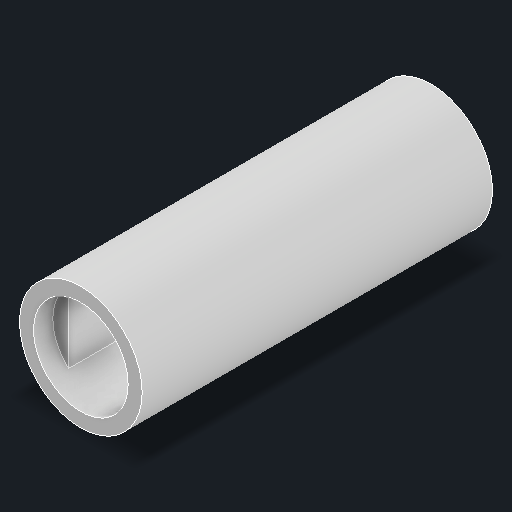
# Autodesk Inventor part: Motor_Lego_Axle_Connector
Saved by Autodesk Inventor 2025 (Build 290162000, 162)
## iProperties
Created: 2024-06-03
Part Number: Motor_Lego_Axle_Connector
Material: Generic
Document SubType Name: Modeling
Designer: Garfieldcmix
Density: 1 g/cm^3
Appearance: Default
Author: Garfieldcmix
Autodesk Inventor part; units mm, degrees
ref_plane "YZ Plane" through (0, 0, 0) normal (1, 0, 0) x (0, 1, 0)
ref_plane "XZ Plane" through (0, 0, 0) normal (0, 1, 0) x (-1, 0, 0)
ref_plane "XY Plane" through (0, 0, 0) normal (0, 0, 1) x (1, 0, 0)
sketch "Motor_Lego_Axle_Connector" plane through (0, 0, 0) normal (0, 0, 1) x (1, 0, 0)
  circle A0 centre (0, 0) radius 3.5
  circle A1 centre (0, 0) radius 2.7
  line L0 (-1.8, 2.0125) -> (-1.8, -2.0125)
  line L1 (0, 3.5) -> (0, -3.5) construction
  line L2 (1.8, 2.0125) -> (1.8, -2.0125)
  line L3 (0.9, 2.4) -> (-0.9, 2.4)
  line L4 (0.9, 2.4) -> (0.9, 1.4)
  line L5 (1.4, 1.4) -> (0.9, 1.4) construction
  line L6 (1.4, 1.4) -> (1.4, 0.9) construction
  arc A2 (0.9, 1.4) -> (1.4, 0.9) centre (1.4, 1.4) ccw
  line L7 (1.4, 0.9) -> (2.4, 0.9)
  line L8 (-0.9, 1.4) -> (-0.9, 2.4)
  arc A3 (-1.4, 0.9) -> (-0.9, 1.4) centre (-1.4, 1.4) ccw
  line L9 (-2.4, 0.9) -> (-1.4, 0.9)
  line L10 (-2.4, 0.9) -> (-2.4, -0.9)
  line L11 (-1.4, -0.9) -> (-2.4, -0.9)
  arc A4 (-0.9, -1.4) -> (-1.4, -0.9) centre (-1.4, -1.4) ccw
  line L12 (-0.9, -2.4) -> (-0.9, -1.4)
  line L13 (-0.9, -2.4) -> (0.9, -2.4)
  line L14 (0.9, -1.4) -> (0.9, -2.4)
  arc A5 (1.4, -0.9) -> (0.9, -1.4) centre (1.4, -1.4) ccw
  line L15 (2.4, -0.9) -> (1.4, -0.9)
  line L16 (2.4, -0.9) -> (2.4, 0.9)
  point P0 (1.8, -2.0125)
  point P1 (0, 2.4)
  point P2 (-2.4, 0)
  point P3 (0, -2.4)
  point P4 (2.4, 0)
  dimension "d0" = 7
  dimension "d1" = 5.4
  dimension "d2" = 7
  dimension "d3" = 1.8
  dimension "d12" = 1.8
  dimension "d13" = 2.4
  dimension "d14" = 1
  dimension "d16" = 0.5
  dimension "d17" = 1
  dimension "d20" = 360
  constraints: 34 end point, 12 point on circle, 6 centre point, 5 perpendicular, 2 coincident, 2 midpoint, 2 symmetric about line, 1 parallel, 1 point on line, 1 vertical, 45 other
  measures "d0" diameter of A0
  measures "d1" diameter of A1
  measures "d2" distance of L1.end L1.start
  measures "d3" distance from line of L0 point (0, 0)
  measures "d12" distance of L3.end L3.start
  measures "d13" distance from line of point (0, 0) L3
  measures "d14" distance of L4.end L3.start
  measures "d16" distance of L4.end L5.start
  measures "d17" distance of L6.end L7.end
extrude "Motor_Side_Outer_Ring_Extrusion" add sketch "Motor_Lego_Axle_Connector" along normal blind 9
extrude "Motor_Connector_Extrusion" add sketch "Motor_Lego_Axle_Connector" along normal blind 7.9 separate body contours A1 L2 L15 L16 L7 | L0 L9 L10 L11 A1 | L7 L16 L15 L2 | L0 L11 L10 L9
extrude "Seperation_Extrusion" add sketch "Motor_Lego_Axle_Connector" against normal blind 3 contours A1 L2 L15 L16 L7 | L2 L7 A2 L4 L3 L8 A3 L9 L0 A1 | A1 L0 L11 A4 L12 L13 L14 A5 L15 L2 | L0 L9 L10 L11 A1 | L7 L16 L15 L2 | L2 L15 A5 L14 L13 L12 A4 L11 L0 L9 A3 L8 L3 L4 A2 L7 | L0 L11 L10 L9
extrude "Lego_Axle_Side_Outer_Ring_Extrusion" add sketch "Motor_Lego_Axle_Connector" against normal blind 11
extrude "Lego_Axle_Connector_Extrusion" add sketch "Motor_Lego_Axle_Connector" against normal blind 11 contours A1 L2 L15 L16 L7 | L2 L7 A2 L4 L3 L8 A3 L9 L0 A1 | A1 L0 L11 A4 L12 L13 L14 A5 L15 L2 | L0 L9 L10 L11 A1
equation "\"d2\" = d0"
body "Solid1"
